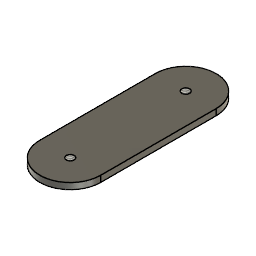
ShellConnector (Autodesk Fusion 360 design; units mm, degrees)
Autodesk Fusion 360 part; units mm, degrees
note: some values were not read from the file. Set by a fixed rule: the direction of a hole.
sketch "Sketch1" plane through (0, 0, 0) normal (0, 0, 1) x (1, 0, 0)
  line L0 (-9.3846, 17.702) -> (-9.3846, -19.298)
  arc A0 (-9.3846, -19.298) -> (10.1154, -19.298) centre (0.3654, -19.298) ccw
  line L1 (10.1154, -19.298) -> (10.1154, 17.702)
  arc A1 (10.1154, 17.702) -> (-9.3846, 17.702) centre (0.3654, 17.702) ccw
  line L2 (0.3654, 17.702) -> (0.3654, -19.298) construction
  dimension "d1" = 37
  dimension "d2" = 9.75
  constraint tangent L0 A0
  constraint tangent A0 L1
  constraint parallel L0 L1
  constraint tangent L1 A1
  constraint tangent L0 A1
  constraint vertical L2
  measures "d1" distance of L0.start L0.end
  measures "d2" radius of A1
extrude "Extrude1" add sketch "Sketch1" along normal blind 2
hole "Hole1" at (0.3654, 17.702, 0) at (0.3654, -19.298, 0) direction (0, 0, 1) diameter 2.529 depth 2 tip angle 180 countersink diameter 2.782 countersink angle 90
thread "Thread1" "ISO Metric profile 3.0 M3x0.5 M3x0.5 6H" thread offset 0 thread depth 7.4
